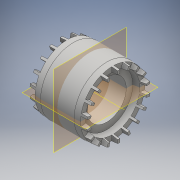
# Autodesk Inventor part: Сердечник ротора
Saved by Autodesk Inventor 2016 SP1 (Build 200210100, 210)
## iProperties
Created: 2016-05-15
Part Number: Сердечник ротора
Material: Типовые
Document SubType Name: Modeling
Designer: AS
Density: 1 g/cm^3
Appearance: По умолчанию
Author: AS
Autodesk Inventor part; units mm, degrees
ref_plane "XZ Plane" through (0, 0, 0) normal (0, 1, 0) x (-1, 0, 0)
sketch "Эскиз1" plane through (0, 0, 0) normal (0, 0, 1) x (1, 0, 0)
  line L0 (-28, -32.5) -> (28, -32.5)
  line L1 (28, -32.5) -> (28, -43.5)
  line L2 (28, -54.5) -> (-28, -54.5)
  line L3 (-28, -43.5) -> (-28, -32.5)
  line L4 (-67.2, 0) -> (67.2, 0) projected
  line L5 (-48, -52.7502) -> (-48, -47.0265)
  line L6 (-28, -43.5) -> (-48, -47.0265)
  line L7 (-28, -54.5) -> (-48, -52.7502)
  line L8 (28, -54.5) -> (48, -52.7502)
  line L9 (28, -43.5) -> (48, -47.0265)
  line L10 (48, -52.7502) -> (48, -47.0265)
  point P0 (0, 0)
  dimension "d0" = 56
  dimension "d1" = 32.5
  dimension "d2" = 22
  dimension "d3" = 28
  dimension "d5" = 20
  dimension "d6" = 5
  dimension "d7" = 10
  dimension "d8" = 20
  dimension "d9" = 5
  dimension "d10" = 10
  dimension "d11" = 28
  dimension "d12" = 22
  dimension "d13" = 11
  dimension "d14" = 11
  constraints: 20 end point, 2 parallel, 2 vertical, 1 horizontal, 1 perpendicular
  measures "d0" distance of L2.start L2.end
  measures "d1" distance from line of L0 point (0, 0)
  measures "d2" distance of L0.end L2.start
  measures "d3" horizontal distance of point (0, 0) L0.start
  measures "d5" distance between parallel lines of L5 L3
  measures "d6" angle of L7 L2
  measures "d7" angle of L6 L0
  measures "d8" distance between parallel lines of L10 L1
  measures "d9" angle of L8 L2
  measures "d10" angle of L9 L0
  measures "d11" distance from line of L1 point (0, 0)
  measures "d12" distance between parallel lines of L2 L0
  measures "d13" distance from line of L3.start L0
  measures "d14" distance of L0.end L1.end
revolve "Вращение1" add sketch "Эскиз1" angle 360 about axis through (-10, 0, 0) along (1, 0, 0)
ref_plane "РабПлоскость1" through (-48, 0, 0) normal (-1, 0, 0) x (0, 0, 1)
sketch "Эскиз3" plane through (-48, 0, 0) normal (-1, 0, 0) x (0, 0, 1)
  circle A0 centre (0, 0) radius 32.5 projected
  arc A1 (-8.6859, -61.8032) -> (8.6859, -61.8032) centre (0, 0) ccw
  line L0 (0, 0) -> (8.6859, -61.8032)
  line L1 (0, 79.8796) -> (0, -97.7775) construction
  line L2 (0, 0) -> (-8.6859, -61.8032)
  point P0 (6.334, -72.3979)
  point P1 (-6.334, -72.3979)
  dimension "d17" = 8
  dimension "d18" = 8
  constraints: 4 end point, 2 point on circle, 1 centre point, 1 coincident, 1 symmetric about line
  measures "d17" angle of L0 L1
  measures "d18" angle of L2 L1
extrude "Выдавливание1" cut sketch "Эскиз3" against normal blind 10 contours L2 L0 A0 | A0 L0 A1 L2 picked at (2.0117, -21.5495)
pattern_circular "Круговой массив1" count 18 over 360 about axis through (-10, 0, 0) along (1, 0, 0) of "Выдавливание1"
ref_plane "РабПлоскость2" through (48, 0, 0) normal (1, 0, 0) x (0, 0, -1)
sketch "Эскиз4" plane through (48, 0, 0) normal (1, 0, 0) x (0, 0, -1)
  circle A0 centre (-0.7714, 0) radius 62.1571
  arc A1 (45.2357, 1.5797) -> (43.0479, 13.9871) centre (0, 0) ccw projected
  line L0 (0, 0) -> (8.635, -61.4412)
  line L1 (0, 0) -> (-8.6649, -61.6539)
  line L2 (0, -87.02) -> (0, 87.02) construction
  dimension "d25" = 8
  dimension "d26" = 8
  constraints: 4 end point, 2 point on circle, 1 centre point
  measures "d25" angle of L0 L2
  measures "d26" angle of L2 L1
extrude "Выдавливание2" cut sketch "Эскиз4" against normal blind 10 contours L1 L0 A0 picked at (-3.855, -41.2582)
pattern_circular "Круговой массив2" count 18 over 360 about axis through (-10, 0, 0) along (1, 0, 0) of "Выдавливание2"
equation "\"d3\" = 0.5 * d0"
equation "\"d8\" = d5"
equation "\"d9\" = d6"
equation "\"d10\" = d7"
equation "\"d11\" = d3"
equation "\"d13\" = 0.5 * d12"
equation "\"d14\" = d13"
equation "\"d18\" = d17"
equation "\"d26\" = d25"
